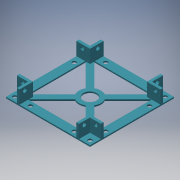
# Autodesk Inventor part: Base
Saved by Autodesk Inventor 2016 (Build 200138000, 138)
## iProperties
Created: 2015-03-29
Part Number: Base
Material: PC/ABS Plastic
Document SubType Name: Modeling
Designer: Erin
Density: 0.357273 g/cm^3
Appearance: Cadet Blue
Mass: 3.14413 g
Surface Area: 66.4965 cm^2
Volume: 5.71659 cm^3
Author: Erin
Autodesk Inventor part; units mm, degrees
ref_plane "YZ Plane" through (0, 0, 0) normal (1, 0, 0) x (0, 1, 0)
ref_plane "XZ Plane" through (0, 0, 0) normal (0, 1, 0) x (-1, 0, 0)
ref_plane "XY Plane" through (0, 0, 0) normal (0, 0, 1) x (1, 0, 0)
sketch "Sketch1" plane through (0, 0, 0) normal (0, 0, 1) x (1, 0, 0)
  line L0 (-48, 48) -> (48, 48)
  line L1 (48, 48) -> (48, -48)
  line L2 (48, -48) -> (-48, -48)
  line L3 (-48, -48) -> (-48, 48)
  line L4 (38, 38) -> (-38, 38)
  line L5 (-38, 38) -> (-38, -38)
  line L6 (-38, -38) -> (38, -38)
  line L7 (38, -38) -> (38, 38)
  line L8 (0, 61.066) -> (0, -72.1628) construction
  line L9 (-77.8847, 0) -> (88.8171, 0) construction
  line L10 (-48, 43) -> (48, 43) construction
  line L11 (-43, 48) -> (-43, -48) construction
  line L12 (-48, -43) -> (48, -43) construction
  circle A0 centre (-43, 25) radius 2.25
  circle A1 centre (-43, -25) radius 2.25
  circle A2 centre (-43, -43) radius 2.25
  circle A3 centre (-43, 43) radius 2.25
  line L13 (-48, 30) -> (48, 30) construction
  line L14 (-48, -30) -> (48, -30) construction
  line L15 (-50, 31) -> (-36, 31)
  line L16 (-36, 31) -> (-36, -31)
  line L17 (-36, -31) -> (-50, -31)
  line L18 (-50, -31) -> (-50, 31)
  point P0 (0, 0)
  point P1 (0, 48)
  point P2 (48, 0)
  dimension "d0" = 96
  dimension "d1" = 96
  dimension "d2" = 10
  dimension "d5" = 5
  dimension "d11" = 5
  dimension "d14" = 5
  dimension "d31" = 4.5
  dimension "d32" = 4.5
  dimension "d61" = 4.5
  dimension "d62" = 4.5
  dimension "d65" = 30
  dimension "d66" = 30
  dimension "d67" = 5
  dimension "d68" = 5
  dimension "d74" = 1
  dimension "d75" = 1
  dimension "d76" = 2
  dimension "d77" = 2
  constraints: 38 end point, 16 point on line, 9 perpendicular, 7 parallel, 4 centre point, 3 horizontal, 2 midpoint, 1 horizontal alignment, 1 vertical, 1 vertical alignment, 3 other
  measures "d0" distance of L1.end L2.end
  measures "d1" distance of L0.end L1.end
  measures "d2" distance between parallel lines of L4 L0
  measures "d5" distance between parallel lines of L10 L0
  measures "d11" distance between parallel lines of L11 L3
  measures "d14" distance between parallel lines of L12 L2
  measures "d31" diameter of A0
  measures "d32" diameter of A1
  measures "d61" diameter of A2
  measures "d62" diameter of A3
  measures "d65" distance between parallel lines of L13 L9
  measures "d66" distance between parallel lines of L14 L9
  measures "d67" distance from line of A1.centre L14
  measures "d68" distance from line of A0.centre L13
  measures "d74" distance between parallel lines of L13 L15
  measures "d75" distance between parallel lines of L17 L14
  measures "d76" distance between parallel lines of L3 L18
  measures "d77" distance between parallel lines of L16 L5
extrude "Extrusion1" add sketch "Sketch1" against normal blind 1.5 contours L0 L1 L2 L3 L17 L5 L6 L7 L4 L15 | L15 L5 L17 L3 | A0 | A1 | A2 | A3
extrude "Extrusion2" cut sketch "Sketch1" against normal blind 10 contours A2 | A3
mirror "Mirror5" about plane through (0, 0, 0) normal (1, 0, 0) of "Extrusion2"
extrude "Extrusion5" cut sketch "Sketch1" against normal blind 10 contours A0 | A1
pattern_circular "Circular Pattern2" count 4 over 360 about axis through (0, 0, -10) along (0, 0, 1) of "Extrusion5"
sketch "Sketch5" plane through (0, 0, 0) normal (0, 0, 1) x (1, 0, 0)
  line L0 (-48, -48) -> (-48, 48) projected
  line L1 (-38, -38) -> (-38, 38) projected
  line L2 (-48, -35.5) -> (-38, -35.5)
  line L3 (-38, -35.5) -> (-38, -32.5)
  line L4 (-38, -32.5) -> (-48, -32.5)
  line L5 (-48, -32.5) -> (-48, -35.5)
  line L6 (-51.6876, -22.75) -> (-34.0834, -22.75)
  line L7 (-34.0834, -22.75) -> (-34.0834, -45.25)
  line L8 (-34.0834, -45.25) -> (-51.6876, -45.25)
  line L9 (-51.6876, -45.25) -> (-51.6876, -22.75)
  circle A0 centre (-43, -25) radius 2.25 projected
  circle A1 centre (-43, -43) radius 2.25 projected
  line L10 (-22.75, -50) -> (-45.25, -50)
  line L11 (-45.25, -50) -> (-45.25, -36.2343)
  line L12 (-45.25, -36.2343) -> (-22.75, -36.2343)
  line L13 (-22.75, -36.2343) -> (-22.75, -50)
  circle A2 centre (-25, -43) radius 2.25 projected
  line L14 (38, -38) -> (-38, -38) projected
  line L15 (48, -48) -> (-48, -48) projected
  line L16 (-32.5, -38) -> (-35.5, -38)
  line L17 (-35.5, -38) -> (-35.5, -48)
  line L18 (-35.5, -48) -> (-32.5, -48)
  line L19 (-32.5, -48) -> (-32.5, -38)
  line L20 (-32.5, -32.5) -> (-38, -32.5)
  line L21 (-38, -32.5) -> (-38, -35.5)
  line L22 (-38, -35.5) -> (-32.5, -35.5)
  line L23 (-32.5, -35.5) -> (-32.5, -32.5)
  line L24 (-32.5, -35.5) -> (-35.5, -35.5)
  line L25 (-35.5, -35.5) -> (-35.5, -38)
  line L26 (-35.5, -38) -> (-32.5, -38)
  line L27 (-32.5, -38) -> (-32.5, -35.5)
  line L28 (-38, -38) -> (-35.5, -38)
  line L29 (-35.5, -38) -> (-35.5, -35.5)
  line L30 (-35.5, -35.5) -> (-38, -35.5)
  line L31 (-38, -35.5) -> (-38, -38)
  point P0 (0, 0)
  point P1 (-38, -34)
  point P2 (-34.0834, -34)
  point P3 (-34, -38)
  point P4 (-34, -36.2343)
  dimension "d95" = 3
  dimension "d96" = 3
  constraints: 56 end point, 14 parallel, 7 horizontal, 7 perpendicular, 4 midpoint, 4 point on line, 4 tangent, 1 horizontal alignment, 1 vertical alignment
  measures "d95" distance of L3.end L2.end
  measures "d96" distance of L18.end L17.end
extrude "Extrusion9" add sketch "Sketch5" along normal blind 15 contours L0 L4 L1 L2 | L1 L20 L7 L22 | L22 L7 L12 L25 | L20 L23 L22 L7 | L12 L7 L14 L25 | L22 L27 L12 L7 | L17 L8 L7 L14 L19 L15 | L17 L14 L7 L8 | L12 L27 L14 L7
extrude "Extrusion10" add sketch "Sketch5" against normal blind 1.5 contours L22 L25 L12 L1 | L1 L20 L7 L22 | L12 L25 L14 L1 | L22 L7 L12 L25 | L20 L23 L22 L7 | L12 L7 L14 L25 | L22 L27 L12 L7 | L12 L27 L14 L7
sketch "Sketch6" plane through (-48, -35.5, 15) normal (0, -1, 0) x (1, 0, 0)
  line L0 (12.5, -15) -> (12.5, 0) projected
  line L1 (0, 0) -> (12.5, 0) projected
  line L2 (0, -15) -> (0, 0) projected
  line L3 (0, -15) -> (12.5, -15) projected
  circle A0 centre (6.25, -4) radius 2.25
  point P0 (48, -15)
  dimension "d101" = 4.5
  dimension "d102" = 4
  constraints: 1 centre point
  measures "d101" diameter of A0
  measures "d102" distance from line of A0.centre L1
extrude "Extrusion11" cut sketch "Sketch6" against normal blind 5 contours A0
sketch "Sketch7" plane through (-35.5, -48, 0) normal (-1, 0, 0) x (0, 0, 1)
  line L0 (0, 12.5) -> (0, 0) projected
  line L1 (0, 0) -> (15, 0) projected
  line L2 (15, 12.5) -> (15, 0) projected
  line L3 (0, 12.5) -> (15, 12.5) projected
  circle A0 centre (11, 6.25) radius 2.25
  point P0 (0, 48)
  dimension "d105" = 4.5
  dimension "d106" = 4
  constraints: 1 centre point
  measures "d105" diameter of A0
  measures "d106" distance from line of A0.centre L2
extrude "Extrusion12" cut sketch "Sketch7" against normal blind 5 contours A0
pattern_circular "Circular Pattern3" count 4 over 360 about axis through (0, 0, -10) along (0, 0, 1) of "Extrusion9", "Extrusion10", "Extrusion11", "Extrusion12"
sketch "Sketch8" plane through (0, 0, 0) normal (0, 0, 1) x (1, 0, 0)
  line L0 (48, 48) -> (48, -48) projected
  line L1 (-48, 48) -> (48, 48) projected
  line L2 (-48, 35.5) -> (-48, 48) projected
  line L3 (-48, -48) -> (-48, 48) projected
  line L4 (48, -48) -> (-48, -48) projected
  circle A0 centre (0, 0) radius 7.5
  circle A1 centre (0, 0) radius 12.5
  line L5 (-40.4749, -35.5251) -> (35.5251, 40.4749)
  line L6 (35.5251, 40.4749) -> (40.4749, 35.5251)
  line L7 (40.4749, 35.5251) -> (-35.5251, -40.4749)
  line L8 (-35.5251, -40.4749) -> (-40.4749, -35.5251)
  line L9 (-38, -38) -> (38, 38) construction
  line L10 (-2.4749, 2.4749) -> (2.4749, -2.4749) construction
  line L11 (-32.5, 38) -> (32.5, 38) projected
  line L12 (38, 38) -> (-38, 38) projected
  line L13 (38, -38) -> (38, 38) projected
  dimension "d112" = 15
  dimension "d113" = 5
  dimension "d114" = 7
  constraints: 12 end point, 5 midpoint, 3 coincident, 2 centre point, 2 parallel, 1 perpendicular
  measures "d112" diameter of A0
  measures "d113" radial gap between concentric circles of A0 A1
  measures "d114" distance of L5.end L6.end
extrude "Extrusion13" add sketch "Sketch8" against normal blind 1.5 contours A0 L7 A1 | A0 L5 A1 L7 | L7 A1 L5 A0 | A0 L5 A1
extrude "Extrusion14" add sketch "Sketch8" against normal blind 1.5 contours L7 A0 L5 | A0 L5 A1 L7 | L7 A1 L5 A0 | A1 L5 L12 L13 L7 | L7 L8 L5 A1 | L13 L6 L7 | L5 L6 L12
mirror "Mirror8" about plane through (0, 0, 0) normal (0, 1, 0) of "Extrusion14"
extrude "Extrusion15" cut sketch "Sketch8" against normal blind 1.5 contours A0 L7 | L7 A0 L5 | L5 A0
equation "\"d31\" = screw"
equation "\"d32\" = screw"
equation "\"d61\" = screw"
equation "\"d62\" = screw"
equation "\"d101\" = screw"
equation "\"d105\" = screw"
equation "\"screw\" = 4.5"
body "Solid1"
